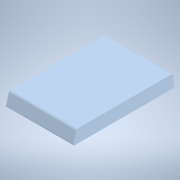
# Autodesk Inventor part: Chassisew
Saved by Autodesk Inventor 2021 (Build 250183000, 183)
## iProperties
Created: 2021-07-24
Part Number: Chassisew
Material: Iron, Gray
Document SubType Name: Modeling
Designer: preet
Density: 7.15 g/cm^3
Appearance: Light Steel Blue
Author: preet
Autodesk Inventor part; units mm, degrees
ref_plane "YZ Plane" through (0, 0, 0) normal (1, 0, 0) x (0, 1, 0)
ref_plane "XZ Plane" through (0, 0, 0) normal (0, 1, 0) x (-1, 0, 0)
ref_plane "XY Plane" through (0, 0, 0) normal (0, 0, 1) x (1, 0, 0)
sketch "Sketch1" plane through (0, 0, 0) normal (1, 0, 0) x (0, 1, 0)
  line L0 (-8.4509, -132.8176) -> (-8.4509, 317.1824)
  line L1 (-8.4509, 317.1824) -> (49.5047, 301.6533)
  line L2 (-8.4509, 317.1824) -> (51.5491, 317.1824) construction
  line L3 (49.5047, 301.6533) -> (49.5047, -128.3467)
  line L4 (49.5047, -128.3467) -> (-8.4509, -132.8176)
  point P0 (0, 0)
  dimension "d0" = 450
  dimension "d1" = 60
  dimension "d2" = 15
  dimension "d3" = 430
  constraints: 10 end point, 2 vertical, 1 equal length, 1 horizontal
  measures "d0" distance of L0.start L0.end
  measures "d1" distance of L0.end L1.end
  measures "d2" angle of L1 L2
  measures "d3" distance of L1.end L3.end
extrude "Extrusion1" add sketch "Sketch1" along normal blind 300
fillet "Fillet1" radius 5 2 edges at (150, -8.4509, 317.1824) (150, -8.4509, -132.8176)
fillet "Fillet2" radius 10 2 edges at (150, 49.5047, 301.6533) (150, 49.5047, -128.3467)
body "Solid1"
